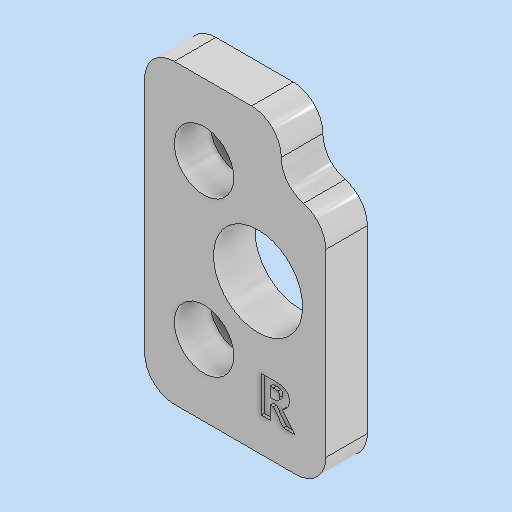
# Autodesk Inventor part: xy Motor Support Right for 4040 extra
Saved by Autodesk Inventor 2023.2 (Build 272271000, 271)
## iProperties
Created: 2024-02-08
Part Number: xy Motor Support Right for 4040 extra
Material: Generisch
Document SubType Name: Modeling
Designer: Nils Bade
Density: 1 g/cm^3
Appearance: Resin-3D-Druck
Description: Fertigung
Auf Bestellliste: True
Author: Nils Bade
Autodesk Inventor part; units mm, degrees
ref_plane "YZ Plane" through (0, 0, 0) normal (1, 0, 0) x (0, 1, 0)
ref_plane "XZ Plane" through (0, 0, 0) normal (0, 1, 0) x (-1, 0, 0)
ref_plane "XY Plane" through (0, 0, 0) normal (0, 0, 1) x (1, 0, 0)
sketch "S-SupportBase" plane through (0, 0, 0) normal (0, 0, 1) x (1, 0, 0)
  line L0 (0, 48) -> (0, -22) construction
  line L1 (0, 0) -> (20.5, 0) construction
  circle A0 centre (0, 0) radius 5
  circle A1 centre (0, 0) radius 3.15
  line L2 (0, -12) -> (20.5, -12)
  line L3 (20.5, -12) -> (20.5, 28)
  line L4 (20.5, 28) -> (13, 28)
  line L5 (13, 28) -> (13, 38)
  line L6 (13, 38) -> (-10, 38)
  line L7 (-10, 38) -> (-10, -12)
  line L8 (-10, -12) -> (0, -12)
  circle A2 centre (0, 26) radius 5
  circle A3 centre (0, 26) radius 3.15
  circle A4 centre (9.0936, 13) radius 7.5
  line L9 (8.9816, -0.1589) -> (15.0717, -0.1589) construction
  line L10 (15.0717, -0.1589) -> (15.0717, -6.2589) construction
  line L11 (15.0717, -6.2589) -> (8.9816, -6.2589) construction
  line L12 (8.9816, -6.2589) -> (8.9816, -0.1589) construction
  line L13 (15.2496, -6.2589) -> (13.386, -6.2589)
  line L14 (13.386, -6.2589) -> (11.6905, -4.0196)
  line L15 (11.6905, -4.0196) -> (11.1368, -4.0196)
  line L16 (11.1368, -4.0196) -> (11.1368, -6.2589)
  line L17 (11.1368, -6.2589) -> (9.6143, -6.2589)
  line L18 (9.6143, -6.2589) -> (9.6143, -0.1589)
  line L19 (9.6143, -0.1589) -> (12.0662, -0.1589)
  spline S0 degree 2 poles (12.0662, -0.1589) (12.5753, -0.1589) (13.3267, -0.2875) (13.648, -0.4852) knots 0 0 0 1 2 2 2
  spline S1 degree 2 poles (13.648, -0.4852) (13.9743, -0.6928) (14.3598, -1.3404) (14.3598, -1.8347) knots 0 0 0 1 2 2 2
  spline S2 degree 2 poles (14.3598, -1.8347) (14.3598, -2.5317) (13.7271, -3.4067) (13.1982, -3.6637) knots 0 0 0 1 2 2 2
  line L20 (13.1982, -3.6637) -> (15.2496, -6.2589)
  spline S3 degree 2 poles (12.7879, -2.0275) (12.7879, -1.7952) (12.6099, -1.464) (12.4072, -1.375) knots 0 0 0 1 2 2 2
  spline S4 degree 2 poles (12.4072, -1.375) (12.2639, -1.3157) (11.9129, -1.2811) (11.6509, -1.2811) knots 0 0 0 1 2 2 2
  line L21 (11.6509, -1.2811) -> (11.1368, -1.2811)
  line L22 (11.1368, -1.2811) -> (11.1368, -2.9222)
  line L23 (11.1368, -2.9222) -> (11.5768, -2.9222)
  spline S5 degree 2 poles (11.5768, -2.9222) (11.8931, -2.9222) (12.343, -2.8431) (12.4962, -2.7196) knots 0 0 0 1 2 2 2
  spline S6 degree 2 poles (12.4962, -2.7196) (12.6445, -2.6009) (12.7879, -2.2846) (12.7879, -2.0275) knots 0 0 0 1 2 2 2
  dimension "d0" = 20.5
  dimension "d1" = 10
  dimension "d2" = 6.3
  dimension "d3" = 12
  dimension "d4" = 10
  dimension "d5" = 40
  dimension "d6" = 10
  dimension "d9" = 26
  dimension "d14" = 23
  dimension "d20" = 15
  constraints: 16 end point, 6 perpendicular, 5 centre point, 3 coincident, 3 point on line, 2 horizontal, 1 vertical, 6 other
  measures "d0" distance of L1.start L1.end
  measures "d1" diameter of A0
  measures "d2" diameter of A1
  measures "d3" distance from line of A1.centre L2
  measures "d4" distance from line of L7 A0.centre
  measures "d5" distance of L2.end L3.end
  measures "d6" distance of L4.end L5.end
  measures "d9" distance of A0.centre A2.centre
  measures "d14" distance between parallel lines of L5 L7
  measures "d20" diameter of A4
extrude "Ex-Base1" add sketch "S-SupportBase" along normal blind 1 contours A0 | L8 L7 L6 L5 L4 L3 L2 | A2 | L13 L14 L15 L16 L17 L18 L19 S0 S1 S2 L20 | S6 S5 L23 L22 L21 S4 S3
extrude "Ex-Base2" add sketch "S-SupportBase" along normal blind 7 contours L8 L7 L6 L5 L4 L3 L2 | L13 L14 L15 L16 L17 L18 L19 S0 S1 S2 L20 | S6 S5 L23 L22 L21 S4 S3
fillet "Rundung1" radius 5 6 edges at (-10, -12, 3.5) (-10, 38, 3.5) (13, 38, 3.5) (13, 28, 3.5) (20.5, 28, 3.5) (20.5, -12, 3.5)
extrude "Extrusion3" cut sketch "S-SupportBase" against normal blind 0.5 from surface at 7 contours L13 L14 L15 L16 L17 L18 L19 S0 S1 S2 L20
